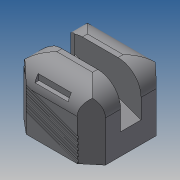
# Autodesk Inventor part: Robot1_A
Saved by Autodesk Inventor 2015 SP1 (Build 190203100, 203)
## iProperties
Created: 2014-10-25
Part Number: Robot1_A
Material: Generic
Document SubType Name: Modeling
Designer: Flopy
Density: 1 g/cm^3
Appearance: Default
Author: Flopy
Autodesk Inventor part; units mm, degrees
ref_plane "YZ Plane" through (0, 0, 0) normal (1, 0, 0) x (0, 1, 0)
ref_plane "XZ Plane" through (0, 0, 0) normal (0, 1, 0) x (-1, 0, 0)
ref_plane "XY Plane" through (0, 0, 0) normal (0, 0, 1) x (1, 0, 0)
sketch "Sketch1" plane through (0, 0, 0) normal (0, 1, 0) x (-1, 0, 0)
  line L0 (160, -99.654) -> (160, 99.654)
  line L1 (160, 99.654) -> (100, 150)
  line L2 (100, 150) -> (-100, 150)
  line L3 (-100, 150) -> (-160, 99.654)
  line L4 (-160, 99.654) -> (-160, -99.654)
  line L5 (-160, -99.654) -> (-100, -150)
  line L6 (-100, -150) -> (100, -150)
  line L7 (100, -150) -> (160, -99.654)
  line L8 (0, 0) -> (0, 1111.9138) construction
  point P0 (160, 0)
  point P1 (0, -150)
  dimension "d0" = 300
  dimension "d1" = 320
  dimension "d3" = 40
  dimension "d4" = 40
  dimension "d5" = 40
  dimension "d6" = 40
  dimension "d7" = 60
  dimension "d8" = 200
  dimension "d9" = 78.3244
  dimension "d10" = 199.308
  dimension "d30" = 1111.9138
  constraints: 18 end point, 3 equal length, 2 midpoint, 2 parallel, 2 vertical, 1 horizontal alignment, 1 perpendicular, 1 vertical alignment
  measures "d0" distance between parallel lines of L2 L6
  measures "d1" distance between parallel lines of L4 L0
  measures "d3" angle of L6 L7
  measures "d4" angle of L2 L1
  measures "d5" angle of L2 L3
  measures "d6" angle of L5 L6
  measures "d7" distance from line of L2.end L4
  measures "d8" distance of L5.end L6.end
  measures "d9" distance of L4.end L5.end
  measures "d10" distance of L3.end L4.end
  measures "d30" distance of L8.start L8.end
extrude "Extrusion1" add sketch "Sketch1" along normal blind 250
sketch "Sketch4" plane through (0, 250, 0) normal (0, 1, 0) x (1, 0, 0)
  line L0 (-160, 99.654) -> (-160, -99.654) projected
  line L1 (-160, 85) -> (-100, 25)
  line L2 (-100, 25) -> (-100, -25)
  line L3 (-100, -25) -> (-160, -85)
  point P0 (0, 0)
  point P1 (-100, 0)
  dimension "d31" = 60
  dimension "d32" = 50
  dimension "d33" = 45
  dimension "d34" = 45
  constraints: 6 end point, 2 point on line, 1 horizontal alignment, 1 midpoint, 1 parallel
  measures "d31" distance between parallel lines of L0 L2
  measures "d32" distance of L1.end L2.end
  measures "d33" angle of L2 L1
  measures "d34" angle of L2 L3
extrude "Extrusion3" cut sketch "Sketch4" against normal through all
sketch "Sketch5" plane through (160, 0, 99.654) normal (1, 0, 0) x (0, 0, -1)
  line L0 (-50.346, 0) -> (-50.346, 250) construction
  arc A0 (39.654, 250) -> (-50.346, 160) centre (39.654, 160) ccw
  line L1 (74.654, 250) -> (14.654, 250) construction
  line L2 (14.654, 250) -> (0, 250) construction
  line L3 (0, 250) -> (-50.346, 250) construction
  line L4 (-50.346, 250) -> (0, 250) construction
  line L5 (0, 250) -> (199.308, 250) construction
  line L6 (199.308, 250) -> (249.654, 250) construction
  line L7 (249.654, 250) -> (199.308, 250) construction
  line L8 (199.308, 250) -> (184.654, 250) construction
  line L9 (184.654, 250) -> (124.654, 250) construction
  line L10 (124.654, 250) -> (74.654, 250) construction
  line L11 (0, 250) -> (199.308, 250) construction
  line L12 (-50.346, 160) -> (-50.346, 250)
  line L13 (-50.346, 250) -> (39.654, 250)
  point P0 (99.654, 0)
  dimension "d37" = 90
  constraints: 4 end point, 3 point on circle, 2 point on line, 2 tangent, 1 centre point, 1 perpendicular, 3 other
  measures "d37" radius of A0
extrude "Extrusion4" cut sketch "Sketch5" against normal through all
sketch "Sketch6" plane through (-100, 0, 150) normal (0, 0, 1) x (1, 0, 0)
  line L0 (30, 212.5) -> (160, 212.5)
  line L1 (160, 212.5) -> (160, 187.5)
  line L2 (160, 187.5) -> (30, 187.5)
  line L3 (30, 187.5) -> (30, 212.5)
  line L4 (30, 200) -> (160, 200) construction
  line L5 (0, 0) -> (200, 0) construction
  line L6 (-60, 0) -> (-60, 240.7933) construction
  point P0 (100, 0)
  dimension "d43" = 200
  dimension "d44" = 25
  dimension "d45" = 130
  dimension "d46" = 90
  constraints: 10 end point, 2 midpoint, 2 parallel, 1 horizontal, 1 perpendicular
  measures "d43" distance between parallel lines of L5 L4
  measures "d44" distance of L2.end L0.start
  measures "d45" distance of L1.end L2.end
  measures "d46" distance from line of L4.start L6
extrude "Extrusion5" cut sketch "Sketch6" against normal blind 20
sketch "Sketch7" plane through (-100, 0, 150) normal (0, 0, 1) x (1, 0, 0)
  arc A0 (30, 250) -> (-60, 160) centre (30, 160) ccw
  line L0 (-60, 160) -> (-60, 250)
  line L1 (-60, 250) -> (30, 250)
  line L2 (-35, 250) -> (260, 250) projected
  line L3 (-60, 0) -> (-60, 240.7933) projected
  line L4 (170, 250) -> (260, 250)
  line L5 (260, 250) -> (260, 160)
  arc A1 (260, 160) -> (170, 250) centre (170, 160) ccw
  point P0 (100, 0)
  dimension "d49" = 90
  dimension "d50" = 90
  constraints: 8 end point, 4 point on circle, 4 tangent, 2 centre point, 2 horizontal, 2 point on line, 1 perpendicular, 1 vertical
  measures "d49" radius of A0
  measures "d50" radius of A1
extrude "Extrusion6" cut sketch "Sketch7" against normal through all
mirror "Mirror1" about plane through (0, 0, 0) normal (0, 0, 1) of "Extrusion4", "Extrusion5"
sketch "Sketch8" plane through (0, 0, 0) normal (0, 0, 1) x (1, 0, 0)
  line L0 (-160, 250) -> (-160, 200)
  line L1 (-160, 200) -> (160, 83.5295)
  line L2 (160, 83.5295) -> (160, 250)
  line L3 (160, 250) -> (-160, 250)
  line L4 (70, 250) -> (-70, 250) projected
  line L5 (-160, 0) -> (-160, 160) projected
  line L6 (160, 0) -> (160, 160) projected
  line L7 (100, 0) -> (-100, 0) projected
  point P0 (0, 0)
  dimension "d53" = 20
  dimension "d54" = 200
  constraints: 8 end point, 3 collinear, 1 parallel, 1 vertical
  measures "d53" angle of L7 L1
  measures "d54" distance from line of L7 L0.end
extrude "Extrusion7" cut sketch "Sketch8" along normal mid plane 80
sketch "Sketch9" plane through (-100, 0, 150) normal (0, 0, 1) x (1, 0, 0)
  line L0 (-63.4202, 100) -> (336.5798, -45.5881)
  line L1 (336.5798, -45.5881) -> (340, -36.1912)
  line L2 (340, -36.1912) -> (-60, 109.3969)
  line L3 (-60, 109.3969) -> (-63.4202, 100)
  line L4 (0, 0) -> (200, 0) projected
  line L5 (-60, 0) -> (-60, 160) projected
  point P0 (100, 0)
  dimension "d57" = 10
  dimension "d58" = 20
  dimension "d59" = 400
  dimension "d60" = 100
  constraints: 8 end point, 2 perpendicular, 1 point on line
  measures "d57" distance between parallel lines of L0 L2
  measures "d58" angle of L4 L0
  measures "d59" horizontal distance of L0.start L0.end
  measures "d60" distance from line of L4 L0.start
extrude "Extrusion8" cut sketch "Sketch9" against normal blind 2
pattern_linear "Rectangular Pattern1" count 5 spacing 20 along (0, 1, 0) of "Extrusion8"
mirror "Mirror2" about plane through (0, 0, 0) normal (0, 0, 1) of "Extrusion8", "Rectangular Pattern1"
sketch "Sketch10" plane through (-100, 160, 150) normal (0, 0, 1) x (1, 0, 0)
  line L0 (-130, 17.5) -> (-30, 17.5)
  line L1 (-30, 17.5) -> (-30, 42.5)
  line L2 (-30, 42.5) -> (-130, 42.5)
  line L3 (-130, 42.5) -> (-130, 17.5)
  line L4 (-30, 30) -> (-130, 30) construction
  line L5 (0, -160) -> (200, -160) construction
  line L6 (-60, -160) -> (-60, 0) construction
  point P0 (100, -160)
  dimension "d66" = 190
  dimension "d67" = 25
  dimension "d68" = 30
  dimension "d69" = 100
  constraints: 10 end point, 2 midpoint, 2 parallel, 1 horizontal, 1 perpendicular
  measures "d66" distance between parallel lines of L4 L5
  measures "d67" distance of L2.end L0.start
  measures "d68" distance between parallel lines of L6 L1
  measures "d69" distance of L0.start L0.end
extrude "Extrusion9" cut sketch "Sketch10" against normal through all
sketch "Sketch11" plane through (0, 250, 0) normal (0, 1, 0) x (1, 0, 0)
  circle A0 centre (-130, 0) radius 50
  point P0 (0, 0)
  dimension "d72" = 100
  dimension "d73" = 130
  constraints: 1 centre point, 1 horizontal alignment
  measures "d72" diameter of A0
  measures "d73" distance of point (0, 0) A0.centre
extrude "Extrusion10" cut sketch "Sketch11" against normal blind 190
fillet "Fillet1" radius 10 1 edges at (-80, 60, 0)
equation "\"d4\" = d3"
equation "\"d5\" = d3"
equation "\"d6\" = d3"
equation "\"d30\" = perimeter"
equation "\"d34\" = d33"
equation "\"perimeter\" = 4 * d9 + 2 * d10 + 2 * d8"
body "Solid1"
